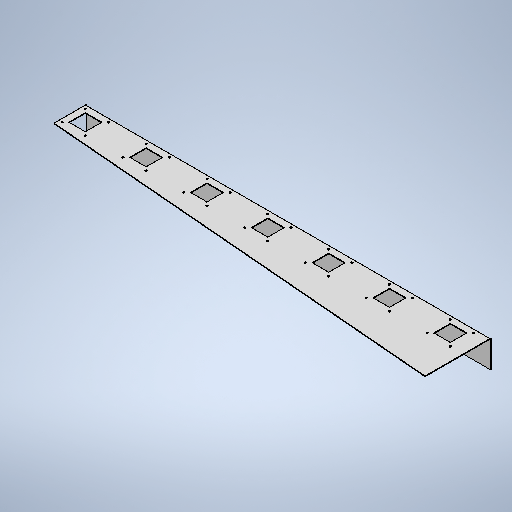
# Autodesk Inventor part: ANP 1422 BOTTOM FDS diameter way up
Saved by Autodesk Inventor 2025.3 (Build 293356030, 356C)
## iProperties
Created: 2024-12-09
Part Number: ANP 1422 BOTTOM FDS diameter way up
Material: Stainless Steel
Document SubType Name: Sheet Metal
Designer: user
Mass: 3269.02 g
Surface Area: 1007.63 cm^2
Volume: 408.627 cm^3
Density: 8 g/cm^3
Flat Pattern Width: 28.2202 cm
Flat Pattern Length: 123 cm
Flat Pattern Area: 3471.08 cm^2
Sheet Metal Rule: AISI304 2mm Die16
Sheet Metal Width: 282,202 mm
Sheet Metal Length: 1230,000 mm
Sheet Metal Area: 347108,449 mm^2
Appearance: Default
Author: user
Autodesk Inventor part; units mm, degrees
ref_plane "YZ Plane" through (0, 0, 0) normal (1, 0, 0) x (0, 1, 0)
ref_plane "XZ Plane" through (0, 0, 0) normal (0, 1, 0) x (-1, 0, 0)
ref_plane "XY Plane" through (0, 0, 0) normal (0, 0, 1) x (1, 0, 0)
sketch "Sketch1" plane through (0, 0, 0) normal (0, 0, 1) x (1, 0, 0)
  line L0 (700, 101) -> (-700, 101)
  line L1 (-700, 101) -> (-700, -101) construction
  line L2 (-700, -101) -> (700, -101) construction
  line L3 (700, -101) -> (700, 101)
  line L4 (700, 101) -> (-700, -101) construction
  line L5 (-700, 101) -> (700, -101) construction
  line L6 (-530, 101) -> (-530, 1)
  line L7 (-530, 1) -> (700, -101)
  point P0 (0, 0)
  point P1 (0, 0)
  point P2 (700, 0)
  dimension "d32" = 202
  dimension "d33" = 1400
  dimension "d60" = 100
  dimension "d61" = 1230
  measures "d32" distance of L2.end L0.start
  measures "d33" distance of L1.end L2.end
  measures "d60" distance of L6.start L6.end
  measures "d61" distance between parallel lines of L3 L6
extrude "Plate1" add sketch "Sketch1" along normal blind 2
sketch "Sketch8" plane through (0, 0, 2) normal (0, 0, 1) x (1, 0, 0)
  line L0 (650, 26) -> (600, 26)
  line L1 (600, 26) -> (600, 76)
  line L2 (600, 76) -> (650, 76)
  line L3 (650, 76) -> (650, 26)
  line L4 (650, 26) -> (600, 76) construction
  line L5 (600, 26) -> (650, 76) construction
  circle A0 centre (660.3553, 15.6447) radius 2.75
  circle A1 centre (589.6447, 15.6447) radius 2.75
  circle A2 centre (589.6447, 86.3553) radius 2.75
  circle A3 centre (660.3553, 86.3553) radius 2.75
  circle A4 centre (625, 51) radius 50 construction
  line L6 (700, 101) -> (700, -101) projected
  line L7 (-530, 101) -> (700, 101) projected
  point P0 (0, 0)
  dimension "d51" = 50
  dimension "d52" = 50
  dimension "d53" = 5.5
  dimension "d54" = 100
  dimension "d72" = 75
  dimension "d73" = 50
  constraints: 12 end point, 5 centre point, 4 point on circle, 4 point on line, 3 equal radius, 2 midpoint, 2 parallel, 1 coincident, 1 horizontal, 1 perpendicular
  measures "d51" distance of L0.start L0.end
  measures "d52" distance of L0.end L1.end
  measures "d53" diameter of A0
  measures "d54" diameter of A4
  measures "d72" distance from line of L6 point (625, 51)
  measures "d73" distance from line of point (625, 51) L7
extrude "Cut3" cut sketch "Sketch8" against normal blind 2
pattern_linear "Rectangular Pattern1" count 7 spacing 185 along (-1, 0, 0) of "Cut3"
sketch "Sketch9" plane through (700, 99, 2) normal (0, 1, 0) x (-1, 0, 0)
  line L0 (1230, 0) -> (0, 0)
  line L1 (0, 0) -> (0, -84)
  line L2 (0, -84) -> (1230, -84)
  line L3 (1230, -84) -> (1230, 0)
  constraints: 6 end point, 1 horizontal, 1 perpendicular, 1 vertical
edge flange "Flange3" height 84 angle 90 thickness 2 bend radius 2.75 thickness toward (0, 1, 0) relief round relief width 2 relief depth 1 edges at (85, 101, 0) wall of the first edge with corners at (-530, 99, 2) (700, 99, 2) (700, 99, -82) (-530, 99, -82)
bend "Bend3"
corner "Corner3"
equation "\"d32\" = MAIN_6_central_window_hight + Thickness"
equation "\"d55\" = Thickness"
equation "\"d2\" = Thickness"
equation "\"d62\" = BendReliefWidth"
equation "\"d63\" = BendReliefDepth"
equation "\"d64\" = MinimumRemnant"
equation "\"d65\" = TransitionRadius"
equation "\"d66\" = MAIN_7_central_window_width + 2 * Thickness"
equation "\"d68\" = BendRadius"
equation "\"d69\" = CornerReliefSize"
equation "\"d70\" = GapSize"
equation "\"d71\" = JacobiRadiusSize"
equation "\"BendReliefWidth\" = Thickness"
equation "\"BendReliefDepth\" = 0.5 * Thickness"
equation "\"CornerReliefSize\" = 4 * Thickness"
equation "\"MinimumRemnant\" = 2 * Thickness"
equation "\"TransitionRadius\" = BendRadius"
equation "\"JacobiRadiusSize\" = BendRadius"
equation "\"GapSize\" = Thickness"
equation "\"MAIN_6_central_window_hight\" = 200"
equation "\"Thickness\" = 2"
equation "\"MAIN_7_central_window_width\" = 80"
equation "\"BendRadius\" = 2.75"
body "Solid1"
